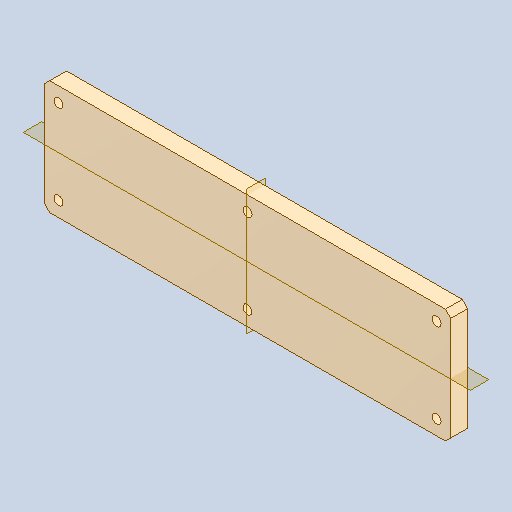
# Autodesk Inventor part: Rear Armor
Saved by Autodesk Inventor 2022 (Build 260153000, 153)
## iProperties
Created: 2022-08-21
Part Number: Rear Armor
Material: Polyethylene, High Density
Document SubType Name: Modeling
Designer: Nick
Density: 0.952 g/cm^3
Appearance: Smooth - Off-White
Mass: 39.723 g
Surface Area: 156.014 cm^2
Volume: 41.7259 cm^3
Author: Nick
Autodesk Inventor part; units mm, degrees
ref_plane "YZ Plane" through (0, 0, 0) normal (1, 0, 0) x (0, 1, 0)
ref_plane "XZ Plane" through (0, 0, 0) normal (0, 1, 0) x (-1, 0, 0)
ref_plane "XY Plane" through (0, 0, 0) normal (0, 0, 1) x (1, 0, 0)
sketch "Sketch1" plane through (0, 0, 0) normal (0, 0, 1) x (1, 0, 0)
  line L0 (0, 0) -> (153, 0)
  line L1 (153, 0) -> (153, 43)
  line L2 (153, 43) -> (0, 43)
  line L3 (0, 43) -> (0, 0)
  dimension "d0" = 43
  dimension "d1" = 153
  constraints: 8 end point, 2 parallel, 1 horizontal, 1 perpendicular
  measures "d0" distance of L2.end L0.start
  measures "d1" distance of L0.start L0.end
extrude "Extrusion1" add sketch "Sketch1" along normal blind 6.35
chamfer "Chamfer1" distance 2 angle 45 4 edges at (0, 43, 3.175) (0, 0, 3.175) (153, 43, 3.175) (153, 0, 3.175)
ref_plane "Work Plane1" through (2, 21.5, 0) normal (0, 1, 0) x (1, 0, 0)
ref_plane "Work Plane2" through (76.5, 2, 0) normal (1, 0, 0) x (0, 0, -1)
sketch "Sketch2" plane through (0, 0, 6.35) normal (0, 0, 1) x (1, 0, 0)
  line L0 (137.7, 37.4031) -> (143.5031, 31.6) projected
  line L1 (149.525, 31.6) -> (143.5031, 31.6) projected
  line L2 (152.7, 34.775) -> (149.525, 31.6) projected
  line L3 (152.7, 43.2063) -> (152.7, 34.775) projected
  line L4 (152.7, 43.2063) -> (0.3, 43.2063) projected
  line L5 (0.3, 34.775) -> (0.3, 43.2063) projected
  line L6 (3.475, 31.6) -> (0.3, 34.775) projected
  line L7 (9.4969, 31.6) -> (3.475, 31.6) projected
  line L8 (9.4969, 31.6) -> (15.3, 37.4031) projected
  line L9 (15.3, 37.4031) -> (66.5, 37.4031) projected
  line L10 (66.5, 37.4031) -> (72.3031, 31.6) projected
  line L11 (80.6969, 31.6) -> (72.3031, 31.6) projected
  line L12 (80.6969, 31.6) -> (86.5, 37.4031) projected
  line L13 (86.5, 37.4031) -> (137.7, 37.4031) projected
  circle A0 centre (76.5, 37.4031) radius 1.7018 projected
  circle A1 centre (147.7, 37.4031) radius 1.7018 projected
  circle A2 centre (5.3, 37.4031) radius 1.7018 projected
  line L14 (15.27, 5.5969) -> (9.4669, 11.4) projected
  line L15 (3.445, 11.4) -> (9.4669, 11.4) projected
  line L16 (0.27, 8.225) -> (3.445, 11.4) projected
  line L17 (0.27, -0.2063) -> (0.27, 8.225) projected
  line L18 (0.27, -0.2063) -> (152.67, -0.2063) projected
  line L19 (152.67, 8.225) -> (152.67, -0.2063) projected
  line L20 (149.495, 11.4) -> (152.67, 8.225) projected
  line L21 (143.4731, 11.4) -> (149.495, 11.4) projected
  line L22 (143.4731, 11.4) -> (137.67, 5.5969) projected
  line L23 (137.67, 5.5969) -> (86.47, 5.5969) projected
  line L24 (86.47, 5.5969) -> (80.6669, 11.4) projected
  line L25 (72.2731, 11.4) -> (80.6669, 11.4) projected
  line L26 (72.2731, 11.4) -> (66.47, 5.5969) projected
  line L27 (66.47, 5.5969) -> (15.27, 5.5969) projected
  circle A3 centre (76.47, 5.5969) radius 1.7018 projected
  circle A4 centre (5.27, 5.5969) radius 1.7018 projected
  circle A5 centre (147.67, 5.5969) radius 1.7018 projected
  point P0 (0, 0)
  point P1 (76.47, 5.5969)
  point P2 (5.27, 5.5969)
  point P3 (147.67, 5.5969)
hole "Hole1" at (147.7, 37.4031, 6.35) at (76.5, 37.4031, 6.35) at (5.3, 37.4031, 6.35) at (5.27, 5.5969, 6.35) at (76.47, 5.5969, 6.35) at (147.67, 5.5969, 6.35) direction (0, 0, -1) diameter 3.4 depth 8 tip angle 118 clearance for "Flat Head Machine Screw" size "M3" standard "Ansi Metric M Profile"
body "Solid1"
